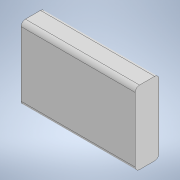
# Autodesk Inventor part: battery_mockup
Saved by Autodesk Inventor 2021 (Build 250183000, 183)
## iProperties
Created: 2024-04-23
Part Number: battery_mockup
Material: Generic
Document SubType Name: Modeling
Designer: Toby
Density: 1 g/cm^3
Appearance: Default
Author: Toby
Autodesk Inventor part; units mm, degrees
ref_plane "YZ Plane" through (0, 0, 0) normal (1, 0, 0) x (0, 1, 0)
ref_plane "XZ Plane" through (0, 0, 0) normal (0, 1, 0) x (-1, 0, 0)
ref_plane "XY Plane" through (0, 0, 0) normal (0, 0, 1) x (1, 0, 0)
sketch "Sketch1" plane through (0, 0, 0) normal (0, 0, 1) x (1, 0, 0)
  line L0 (-28.6335, 13.4746) -> (24.3665, 13.4746)
  line L1 (24.3665, 13.4746) -> (24.3665, -20.5254)
  line L2 (24.3665, -20.5254) -> (-28.6335, -20.5254)
  line L3 (-28.6335, -20.5254) -> (-28.6335, 13.4746)
  point P0 (0, 0)
  dimension "d0" = 53
  dimension "d1" = 34
  constraints: 8 end point, 2 parallel, 1 horizontal, 1 perpendicular
  measures "d0" distance of L0.start L0.end
  measures "d1" distance of L2.end L0.start
extrude "Extrusion1" add sketch "Sketch1" along normal blind 11
fillet "Fillet1" radius 2 4 edges at (-2.1335, 13.4746, 11) (-2.1335, 13.4746, 0) (-2.1335, -20.5254, 11) (-2.1335, -20.5254, 0)
body "Solid1"
